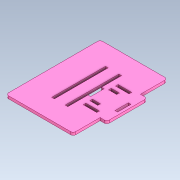
# Autodesk Inventor part: Base
Saved by Autodesk Inventor 2021 (Build 250183000, 183)
## iProperties
Created: 2021-08-28
Part Number: Base
Material: ABS Plastic
Document SubType Name: Modeling
Designer: digge
Density: 1.06 g/cm^3
Appearance: Pink
Author: digge
Autodesk Inventor part; units mm, degrees
ref_plane "YZ Plane" through (0, 0, 0) normal (1, 0, 0) x (0, 1, 0)
ref_plane "XZ Plane" through (0, 0, 0) normal (0, 1, 0) x (-1, 0, 0)
ref_plane "XY Plane" through (0, 0, 0) normal (0, 0, 1) x (1, 0, 0)
sketch "Sketch1" plane through (0, 0, 0) normal (0, 1, 0) x (-1, 0, 0)
  line L0 (104.6154, 153.8462) -> (-145.3846, 153.8462)
  line L1 (-145.3846, 153.8462) -> (-145.3846, -196.1538) construction
  line L2 (-145.3846, -196.1538) -> (104.6154, -196.1538)
  line L3 (104.6154, -196.1538) -> (104.6154, 153.8462)
  line L4 (-20.3846, 153.8462) -> (-20.3846, -196.1538) construction
  line L5 (104.6154, -21.1538) -> (-145.3846, -21.1538) construction
  line L6 (9.6154, 78.8462) -> (-0.3846, 78.8462)
  line L7 (-0.3846, 78.8462) -> (-0.3846, -121.1538)
  line L8 (-0.3846, -121.1538) -> (9.6154, -121.1538)
  line L9 (9.6154, -121.1538) -> (9.6154, 78.8462)
  line L10 (-40.3846, 78.8462) -> (-50.3846, 78.8462)
  line L11 (-50.3846, 78.8462) -> (-50.3846, -121.1538)
  line L12 (-50.3846, -121.1538) -> (-40.3846, -121.1538)
  line L13 (-40.3846, -121.1538) -> (-40.3846, 78.8462)
  line L14 (-145.3846, -196.1538) -> (-145.3846, -96.1538)
  line L15 (-145.3846, 153.8462) -> (-145.3846, 53.8462)
  line L16 (-145.3846, -96.1538) -> (-170.3846, -96.1538)
  line L17 (-170.3846, -96.1538) -> (-170.3846, 53.8462)
  line L18 (-170.3846, 53.8462) -> (-145.3846, 53.8462)
  point P0 (0, 0)
  dimension "d0" = 250
  dimension "d1" = 350
  dimension "d2" = 10
  dimension "d3" = 10
  dimension "d4" = 200
  dimension "d7" = 40
  dimension "d9" = 150
  dimension "d10" = 25
  constraints: 38 end point, 6 parallel, 5 perpendicular, 4 horizontal, 4 midpoint, 2 collinear, 2 point on line, 1 symmetric about line, 2 other
  measures "d0" distance of L0.start L0.end
  measures "d1" distance of L2.end L0.start
  measures "d2" distance of L10.start L10.end
  measures "d3" distance of L6.start L6.end
  measures "d4" distance of L8.end L6.start
  measures "d7" distance between parallel lines of L13 L7
  measures "d9" distance of L15.end L14.end
  measures "d10" distance of L17.end L15.end
extrude "Extrusion2" add sketch "Sketch1" along normal blind 10
fillet "Fillet2" radius 10 6 edges at (170.3846, 5, 53.8462) (170.3846, 5, -96.1538) (145.3846, 5, 153.8462) (145.3846, 5, -196.1538) (-104.6154, 5, -196.1538) (-104.6154, 5, 153.8462)
sketch "Sketch2" plane through (0, 10, 0) normal (0, 1, 0) x (1, 0, 0)
  line L0 (170.3846, -43.8462) -> (170.3846, 86.1538) projected
  line L1 (50.3846, 121.1538) -> (50.3846, -78.8462) projected
  line L2 (145.3846, -53.8462) -> (160.3846, -53.8462) projected
  line L3 (160.3846, 96.1538) -> (145.3846, 96.1538) projected
  line L4 (170.3846, 21.1538) -> (50.3846, 21.1538) construction
  line L5 (160.3846, -3.8462) -> (150.3846, -3.8462)
  line L6 (150.3846, -3.8462) -> (150.3846, 46.1538)
  line L7 (150.3846, 46.1538) -> (160.3846, 46.1538)
  line L8 (160.3846, 46.1538) -> (160.3846, -3.8462)
  line L9 (122.8846, -43.8462) -> (122.8846, -33.8462)
  line L10 (122.8846, -33.8462) -> (72.8846, -33.8462)
  line L11 (72.8846, -33.8462) -> (72.8846, -43.8462)
  line L12 (72.8846, -43.8462) -> (122.8846, -43.8462)
  line L13 (145.3846, -53.8462) -> (50.3846, -53.8462) construction
  line L14 (145.3846, 96.1538) -> (50.3846, 96.1538) construction
  line L15 (97.8846, -53.8462) -> (97.8846, 96.1538) construction
  line L16 (122.8846, 86.1538) -> (122.8846, 76.1538)
  line L17 (122.8846, 76.1538) -> (72.8846, 76.1538)
  line L18 (72.8846, 76.1538) -> (72.8846, 86.1538)
  line L19 (72.8846, 86.1538) -> (122.8846, 86.1538)
  line L20 (50.3846, 46.1538) -> (60.3846, 46.1538)
  line L21 (60.3846, 46.1538) -> (60.3846, -3.8462)
  line L22 (60.3846, -3.8462) -> (50.3846, -3.8462)
  line L23 (50.3846, -3.8462) -> (50.3846, 46.1538)
  line L24 (92.8992, -1.1414) -> (74.8992, -1.1414) construction
  line L25 (74.8992, -1.1414) -> (74.8992, 43.8586) construction
  line L26 (74.8992, 43.8586) -> (92.8992, 43.8586) construction
  line L27 (92.8992, 43.8586) -> (92.8992, -1.1414) construction
  line L28 (72, -8.8462) -> (102, -8.8462)
  line L29 (102, -8.8462) -> (102, -18.8462)
  line L30 (102, -18.8462) -> (72, -18.8462)
  line L31 (72, -18.8462) -> (72, -8.8462)
  line L32 (74.8992, -1.5509) -> (92.8992, -1.5509) construction
  line L33 (72, 51.1538) -> (102, 51.1538)
  line L34 (102, 51.1538) -> (102, 61.1538)
  line L35 (102, 61.1538) -> (72, 61.1538)
  line L36 (72, 61.1538) -> (72, 51.1538)
  point P0 (0, 0)
  point P1 (77.0846, 21.1538)
  dimension "d14" = 26.7
  dimension "d15" = 10
  dimension "d16" = 50
  dimension "d17" = 10
  dimension "d18" = 50
  dimension "d19" = 10
  dimension "d20" = 45
  dimension "d21" = 18
  dimension "d22" = 10
  dimension "d23" = 30
  dimension "d24" = 30
  constraints: 66 end point, 13 perpendicular, 10 symmetric about line, 5 horizontal, 5 point on line, 4 midpoint, 3 parallel, 2 vertical, 3 other
  measures "d14" distance of L4.end point (77.085, 21.154)
  measures "d15" distance of L5.start L5.end
  measures "d16" distance of L5.end L6.end
  measures "d17" distance of L9.start L9.end
  measures "d18" distance of L9.end L10.end
  measures "d19" distance of L21.end L22.end
  measures "d20" distance of L24.end L25.end
  measures "d21" distance of L25.end L26.end
  measures "d22" distance of L28.end L29.end
  measures "d23" distance from line of L4 L28.end
  measures "d24" distance of L29.end L30.end
extrude "Extrusion3" cut sketch "Sketch2" against normal through all
equation "\"d0\" = BaseDepth"
equation "\"d1\" = BaseLength"
equation "\"d2\" = Width"
equation "\"d3\" = Width"
equation "\"d4\" = SlotLength"
equation "\"d7\" = 4 * Width"
equation "\"d11\" = Width"
equation "\"d15\" = Width"
equation "\"d17\" = Width"
equation "\"d19\" = Width"
equation "\"d22\" = Width"
equation "\"BaseDepth\" = 250"
equation "\"BaseLength\" = 350"
equation "\"Width\" = 10"
equation "\"SlotLength\" = 200"
body "Solid2"
